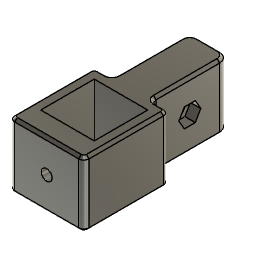
Pin_height_adjuster (Autodesk Fusion 360 design; units mm, degrees)
Autodesk Fusion 360 part; units mm, degrees
sketch "Sketch1" plane through (0, 0, 0) normal (0, 0, 1) x (1, 0, 0)
  line L0 (10, -10) -> (-10, -10)
  line L1 (-10, -10) -> (-10, 10)
  line L2 (-10, 10) -> (10, 10)
  line L3 (10, 10) -> (10, -10)
  line L4 (10, -10) -> (-10, 10) construction
  line L5 (-10, -10) -> (10, 10) construction
  line L6 (10.3, -10.3) -> (-10.3, -10.3)
  line L7 (-10.3, -10.3) -> (-10.3, 10.3)
  line L8 (-10.3, 10.3) -> (10.3, 10.3)
  line L9 (10.3, 10.3) -> (10.3, -10.3)
  line L10 (-14.3, -14.3) -> (-14.3, 14.3)
  line L11 (-14.3, 14.3) -> (14.3, 14.3)
  line L12 (14.3, 14.3) -> (14.3, -14.3)
  line L13 (14.3, -14.3) -> (-14.3, -14.3)
  line L14 (-14.3, -14.3) -> (14.3, -14.3)
  line L15 (14.3, -14.3) -> (14.3, -18.3)
  line L16 (14.3, -18.3) -> (-14.3, -18.3)
  line L17 (-14.3, -18.3) -> (-14.3, -14.3)
  dimension "d1" = 20
  dimension "d2" = 20
  dimension "d3" = -0.3
  dimension "d4" = -4.3
  dimension "d10" = 28.6
  dimension "d11" = 4
  constraint horizontal L0
  constraint perpendicular L0 L1
  constraint parallel L0 L2
  constraint parallel L1 L3
  constraint coincident L4 origin
  constraint coincident L5 origin
  constraint horizontal L14
  constraint vertical L15
  constraint horizontal L16
  constraint vertical L17
  measures "d1" distance of L1.end L2.end
  measures "d2" distance of L0.end L1.end
  measures "d10" distance of L10.start L12.end
  measures "d11" distance of L10.start L16.end
extrude "Extrude1" add sketch "Sketch1" along normal blind 25 contours L10 L11 L12 L13 L14 | L13 L14 L15 L16 L17
sketch "Sketch3" plane through (0, -10.3, 0) normal (0, 1, 0) x (-1, 0, 0)
  line L0 (-10.3, 0) -> (10.3, 0)
  line L1 (10.3, 0) -> (10.3, 25)
  line L2 (10.3, 25) -> (-10.3, 25)
  line L3 (-10.3, 25) -> (-10.3, 0)
  line L4 (-10.3, 25) -> (10.3, 25)
  line L5 (10.3, 25) -> (10.3, 0)
  line L6 (10.3, 0) -> (-10.3, 0)
  line L7 (-10.3, 0) -> (-10.3, 25)
  line L8 (-10.3, 25) -> (10.3, 0) construction
  line L9 (10.3, 25) -> (-10.3, 0) construction
  line L10 (2.1073, 8.85) -> (4.2147, 12.5)
  line L11 (4.2147, 12.5) -> (2.1073, 16.15)
  line L12 (2.1073, 16.15) -> (-2.1073, 16.15)
  line L13 (-2.1073, 16.15) -> (-4.2147, 12.5)
  line L14 (-4.2147, 12.5) -> (-2.1073, 8.85)
  line L15 (-2.1073, 8.85) -> (2.1073, 8.85)
  circle A0 centre (0, 12.5) radius 2.1
  point P0 (0, 12.5)
  dimension "d12" = 25
  dimension "d13" = 3.65
  dimension "d16" = 4.2
  constraint horizontal L4
  constraint vertical L5
  constraint horizontal L6
  constraint vertical L7
  constraint coincident L2.end L3.start
  constraint coincident L0.end L1.start
  constraint midpoint L9 P0
  constraint coincident P0 A0.centre
  measures "d12" distance of L2.end L0.start
  measures "d13" distance of P0 L15
  measures "d16" diameter of A0
extrude "Extrude4" cut sketch "Sketch3" against normal blind 8 contours A0
extrude "Extrude3" cut sketch "Sketch3" against normal blind 4 contours L10 L11 L12 L13 L14 L15 | A0
sketch "Sketch6" plane through (0, 14.3, 0) normal (0, 1, 0) x (-1, 0, 0)
  line L0 (-14.3, 0) -> (14.3, 0)
  line L1 (14.3, 0) -> (14.3, 25)
  line L2 (14.3, 25) -> (-14.3, 25)
  line L3 (-14.3, 25) -> (-14.3, 0)
  line L4 (-14.3, 25) -> (14.3, 0) construction
  line L5 (14.3, 25) -> (-14.3, 0) construction
  line L6 (7.5, 25) -> (-7.5, 25)
  line L7 (-7.5, 25) -> (-7.5, 0)
  line L8 (-7.5, 0) -> (7.5, 0)
  line L9 (7.5, 0) -> (7.5, 25)
  line L10 (7.5, 25) -> (-7.5, 0) construction
  line L11 (-7.5, 25) -> (7.5, 0) construction
  point P0 (0, 12.5)
  dimension "d35" = 15
  dimension "d36" = 25
  constraint coincident L2.end L3.start
  constraint coincident L0.end L1.start
  constraint coincident L1.end L2.start
  constraint coincident L0.start L3.end
  constraint horizontal L6
  constraint perpendicular L6 L7
  constraint parallel L6 L8
  constraint parallel L7 L9
  constraint coincident L10 P0
  constraint coincident L11 P0
  constraint midpoint L5 P0
  measures "d35" distance of L7.end L8.end
  measures "d36" distance of L6.end L7.end
extrude "Extrude10" add sketch "Sketch6" along normal blind 30 contours L0 L2 L6 L7 L8 L9
sketch "Sketch7" plane through (-7.5, 0, 0) normal (-1, 0, 0) x (0, -1, 0)
  line L0 (-14.3, 0) -> (-14.3, 25)
  line L1 (-14.3, 25) -> (-44.3, 25)
  line L2 (-44.3, 25) -> (-44.3, 0)
  line L3 (-44.3, 0) -> (-14.3, 0)
  line L4 (-14.3, 25) -> (-44.3, 0) construction
  line L5 (-44.3, 25) -> (-14.3, 0) construction
  circle A0 centre (-29.3, 12.5) radius 2.1
  line L6 (-27.1927, 8.85) -> (-25.0853, 12.5)
  line L7 (-25.0853, 12.5) -> (-27.1927, 16.15)
  line L8 (-27.1927, 16.15) -> (-31.4073, 16.15)
  line L9 (-31.4073, 16.15) -> (-33.5147, 12.5)
  line L10 (-33.5147, 12.5) -> (-31.4073, 8.85)
  line L11 (-31.4073, 8.85) -> (-27.1927, 8.85)
  line L12 (-29.3, 5.75) -> (-23.4543, 9.125)
  line L13 (-23.4543, 9.125) -> (-23.4543, 15.875)
  line L14 (-23.4543, 15.875) -> (-29.3, 19.25)
  line L15 (-29.3, 19.25) -> (-35.1457, 15.875)
  line L16 (-35.1457, 15.875) -> (-35.1457, 9.125)
  line L17 (-35.1457, 9.125) -> (-29.3, 5.75)
  line L18 (-24.4543, 15.2976) -> (-29.3, 18.0953)
  line L19 (-29.3, 18.0953) -> (-34.1457, 15.2976)
  line L20 (-34.1457, 15.2976) -> (-34.1457, 9.7024)
  line L21 (-34.1457, 9.7024) -> (-29.3, 6.9047)
  line L22 (-29.3, 6.9047) -> (-24.4543, 9.7024)
  line L23 (-24.4543, 9.7024) -> (-24.4543, 15.2976)
  point P0 (-29.3, 12.5)
  point P1 (-29.3, 12.5)
  point P2 (-29.3, 12.5)
  dimension "d43" = 4.2
  dimension "d50" = 3.65
  dimension "d54" = 6.75
  dimension "d55" = -1
  constraint coincident L0.end L1.start
  constraint coincident L2.end L3.start
  constraint coincident L1.end L2.start
  constraint coincident L0.start L3.end
  constraint midpoint L5 P2
  constraint coincident P2 P1
  measures "d43" diameter of A0
  measures "d50" distance of P2 L11
  measures "d54" distance of L12.start P2
extrude "Extrude13" cut sketch "Sketch7" along normal blind 4 from surface at -15 contours L6 L7 L8 L9 L10 L11
extrude "Extrude12" cut sketch "Sketch7" against normal blind 15 contours A0
extrude "Extrude11" add sketch "Sketch7" along normal blind 1.5 contours L12 L13 L14 L15 L16 L17
fillet "Fillet1" radius 3.5 2 edges at (-7.5, 44.3, 12.5) (7.5, 44.3, 12.5)
fillet "Fillet2" radius 2 2 edges at (-7.5, 14.3, 12.5) (7.5, 14.3, 12.5)
fillet "Fillet3" radius 2 4 edges at (-14.3, 14.3, 12.5) (-14.3, -18.3, 12.5) (14.3, -18.3, 12.5) (14.3, 14.3, 12.5)
chamfer "Chamfer1" distance 1 angle 45 32 edges at (-13.7142, -17.7142, 25) (0, -18.3, 25) (13.7142, -17.7142, 25) (14.3, -2, 25) (13.7142, 13.7142, 25) (10.9, 14.3, 25) (8.0858, 14.8858, 25) (7.5, 28.55, 25) (6.4749, 43.2749, 25) (0, 44.3, 25) (-6.4749, 43.2749, 25) (-7.5, 28.55, 25) (-8.0858, 14.8858, 25) (-10.9, 14.3, 25) (-13.7142, 13.7142, 25) (-14.3, -2, 25) (-13.7142, 13.7142, 0) (-10.9, 14.3, 0) (-8.0858, 14.8858, 0) (-7.5, 28.55, 0) (-6.4749, 43.2749, 0) (0, 44.3, 0) (6.4749, 43.2749, 0) (7.5, 28.55, 0) (8.0858, 14.8858, 0) (10.9, 14.3, 0) (13.7142, 13.7142, 0) (14.3, -2, 0) (13.7142, -17.7142, 0) (0, -18.3, 0) (-13.7142, -17.7142, 0) (-14.3, -2, 0)
equation "d35 = 28.6 mm - 4 mm - 4 mm - 0.6 mm - 5 mm"
equation "d54 = ( 13.5 / 2 ) * 1 mm"
